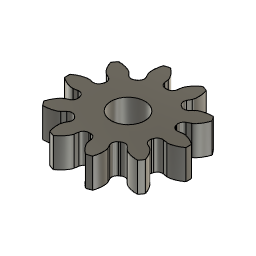
Gearbox Spur Gear (10 teeth) (Autodesk Fusion 360 design; units mm, degrees)
description: Spur Gear; Module: 3.000000; Num Teeth: 10; Pressure Angle: 20.000000; Backlash: 0.15 mm
Autodesk Fusion 360 part; units mm, degrees
sketch "Sketch1" plane through (0, 0, 0) normal (0, 0, 1) x (1, 0, 0)
  circle A0 centre (0, 0) radius 11.3492
  circle A1 centre (0, 0) radius 4
extrude "Extrude1" add sketch "Sketch1" along normal blind 7
sketch "Sketch2" plane through (0, 0, 0) normal (0, 0, 1) x (1, 0, 0)
  spline S0 degree 5 poles (13.8934, -2.3775) (13.905, -2.3795) (13.9281, -2.383) (13.9629, -2.3871) (14.0095, -2.3904) (14.0681, -2.3913) (14.127, -2.39) (14.1859, -2.3873) (14.245, -2.3839) (14.3041, -2.38) (14.3633, -2.3756) (14.4226, -2.3704) (14.4819, -2.3642) (14.5412, -2.3568) (14.6007, -2.3484) (14.6602, -2.339) (14.7197, -2.3287) (14.7792, -2.3176) (14.8387, -2.3059) (14.8983, -2.2936) (14.9578, -2.2807) (15.0174, -2.2671) (15.0769, -2.2528) (15.1365, -2.2378) (15.196, -2.222) (15.2555, -2.2057) (15.3151, -2.1886) (15.3745, -2.171) (15.434, -2.1527) (15.4934, -2.1339) (15.5528, -2.1145) (15.6122, -2.0946) (15.6715, -2.074) (15.7307, -2.0529) (15.79, -2.0312) (15.8491, -2.0089) (15.9083, -1.9861) (15.9673, -1.9627) (16.0263, -1.9388) (16.0853, -1.9144) (16.1442, -1.8894) (16.203, -1.864) (16.2618, -1.838) (16.3204, -1.8115) (16.3791, -1.7844) (16.4376, -1.7569) (16.496, -1.7289) (16.5544, -1.7004) (16.6127, -1.6714) (16.6709, -1.6419) (16.729, -1.6119) (16.787, -1.5814) (16.845, -1.5505) (16.9028, -1.5191) (16.9605, -1.4872) (17.0182, -1.4548) (17.0757, -1.422) (17.1331, -1.3888) (17.1904, -1.355) (17.2477, -1.3208) (17.3048, -1.2862) (17.3618, -1.2511) (17.4186, -1.2156) (17.4754, -1.1796) (17.532, -1.1432) (17.5885, -1.1064) (17.6449, -1.0691) (17.7012, -1.0314) (17.7573, -0.9932) (17.8133, -0.9546) (17.8692, -0.9156) (17.9138, -0.8841) (17.9472, -0.8603) (17.9695, -0.8443) (17.9806, -0.8363) knots 0 0 0 0 0 0 0.01428571 0.02857143 0.04285714 0.05714286 0.07142857 0.08571429 0.1 0.11428571 0.12857143 0.14285714 0.15714286 0.17142857 0.18571429 0.2 0.21428571 0.22857143 0.24285714 0.25714286 0.27142857 0.28571429 0.3 0.31428571 0.32857143 0.34285714 0.35714286 0.37142857 0.38571429 0.4 0.41428571 0.42857143 0.44285714 0.45714286 0.47142857 0.48571429 0.5 0.51428571 0.52857143 0.54285714 0.55714286 0.57142857 0.58571429 0.6 0.61428571 0.62857143 0.64285714 0.65714286 0.67142857 0.68571429 0.7 0.71428571 0.72857143 0.74285714 0.75714286 0.77142857 0.78571429 0.8 0.81428571 0.82857143 0.84285714 0.85714286 0.87142857 0.88571429 0.9 0.91428571 0.92857143 0.94285714 0.95714286 0.97142857 0.98571429 1 1 1 1 1 1
  spline S1 degree 5 poles (13.8934, 2.3775) (13.905, 2.3795) (13.9281, 2.383) (13.9629, 2.3871) (14.0095, 2.3904) (14.0681, 2.3913) (14.127, 2.39) (14.1859, 2.3873) (14.245, 2.3839) (14.3041, 2.38) (14.3633, 2.3756) (14.4226, 2.3704) (14.4819, 2.3642) (14.5412, 2.3568) (14.6007, 2.3484) (14.6602, 2.339) (14.7197, 2.3287) (14.7792, 2.3176) (14.8387, 2.3059) (14.8983, 2.2936) (14.9578, 2.2807) (15.0174, 2.2671) (15.0769, 2.2528) (15.1365, 2.2378) (15.196, 2.222) (15.2555, 2.2057) (15.3151, 2.1886) (15.3745, 2.171) (15.434, 2.1527) (15.4934, 2.1339) (15.5528, 2.1145) (15.6122, 2.0946) (15.6715, 2.074) (15.7307, 2.0529) (15.79, 2.0312) (15.8491, 2.0089) (15.9083, 1.9861) (15.9673, 1.9627) (16.0263, 1.9388) (16.0853, 1.9144) (16.1442, 1.8894) (16.203, 1.864) (16.2618, 1.838) (16.3204, 1.8115) (16.3791, 1.7844) (16.4376, 1.7569) (16.496, 1.7289) (16.5544, 1.7004) (16.6127, 1.6714) (16.6709, 1.6419) (16.729, 1.6119) (16.787, 1.5814) (16.845, 1.5505) (16.9028, 1.5191) (16.9605, 1.4872) (17.0182, 1.4548) (17.0757, 1.422) (17.1331, 1.3888) (17.1904, 1.355) (17.2477, 1.3208) (17.3048, 1.2862) (17.3618, 1.2511) (17.4186, 1.2156) (17.4754, 1.1796) (17.532, 1.1432) (17.5885, 1.1064) (17.6449, 1.0691) (17.7012, 1.0314) (17.7573, 0.9932) (17.8133, 0.9546) (17.8692, 0.9156) (17.9138, 0.8841) (17.9472, 0.8603) (17.9695, 0.8443) (17.9806, 0.8363) knots 0 0 0 0 0 0 0.01428571 0.02857143 0.04285714 0.05714286 0.07142857 0.08571429 0.1 0.11428571 0.12857143 0.14285714 0.15714286 0.17142857 0.18571429 0.2 0.21428571 0.22857143 0.24285714 0.25714286 0.27142857 0.28571429 0.3 0.31428571 0.32857143 0.34285714 0.35714286 0.37142857 0.38571429 0.4 0.41428571 0.42857143 0.44285714 0.45714286 0.47142857 0.48571429 0.5 0.51428571 0.52857143 0.54285714 0.55714286 0.57142857 0.58571429 0.6 0.61428571 0.62857143 0.64285714 0.65714286 0.67142857 0.68571429 0.7 0.71428571 0.72857143 0.74285714 0.75714286 0.77142857 0.78571429 0.8 0.81428571 0.82857143 0.84285714 0.85714286 0.87142857 0.88571429 0.9 0.91428571 0.92857143 0.94285714 0.95714286 0.97142857 0.98571429 1 1 1 1 1 1
  arc A0 (17.9806, -0.8363) -> (17.9806, 0.8363) centre (0, 0) ccw
  line L0 (11.1767, -1.9143) -> (13.8934, -2.3775)
  line L1 (11.1767, 1.9143) -> (13.8934, 2.3775)
  line L2 (11.1767, -1.9143) -> (11.1767, 1.9143)
  point P0 (14.1746, -2.3877)
  point P1 (14.4609, -2.3662)
  point P2 (14.7503, -2.3229)
  point P3 (15.042, -2.2611)
  point P4 (15.3354, -2.1825)
  point P5 (15.6299, -2.0883)
  point P6 (15.9252, -1.9793)
  point P7 (16.2208, -1.856)
  point P8 (16.5163, -1.7189)
  point P9 (16.8114, -1.5683)
  point P10 (17.1057, -1.4046)
  point P11 (17.3989, -1.2278)
  point P12 (17.6907, -1.0383)
  point P13 (14.1746, 2.3877)
  point P14 (14.4609, 2.3662)
  point P15 (14.7503, 2.3229)
  point P16 (15.042, 2.2611)
  point P17 (15.3354, 2.1825)
  point P18 (15.6299, 2.0883)
  point P19 (15.9252, 1.9793)
  point P20 (16.2208, 1.856)
  point P21 (16.5163, 1.7189)
  point P22 (16.8114, 1.5683)
  point P23 (17.1057, 1.4046)
  point P24 (17.3989, 1.2278)
  point P25 (17.6907, 1.0383)
extrude "Extrude2" add sketch "Sketch2" along normal blind 7
fillet "Fillet1" radius 1.5875 2 edges at (11.1863, -1.9159, 3.5) (11.1863, 1.9159, 3.5)
pattern_circular "C-Pattern1" count 10 over 360 about axis through (0, 0, 0) along (0, 0, 1) of "Extrude2", "Fillet1"
sketch "Sketch3" plane through (0, 0, 0) normal (0, 0, 1) x (1, 0, 0)
  circle A0 centre (0, 0) radius 15 construction
scale "Scale1" factor 0.8 about (4.761, 17.359, 7) bodies 1
sketch "sketch 1143" plane through (0, 0, 7) normal (0, 0, 1) x (-1, 0, 0)
  circle A0 centre (-0.9522, -3.4718) radius 3.2
  circle A1 centre (-0.9522, -3.4718) radius 4
extrude "Extrude3" cut sketch "sketch 1143" against normal blind 8
extrude "Extrude4" add 1 faces at (8.2591, 3.4718, 1.4) along direction (0, 0, -1) blind 1.4
